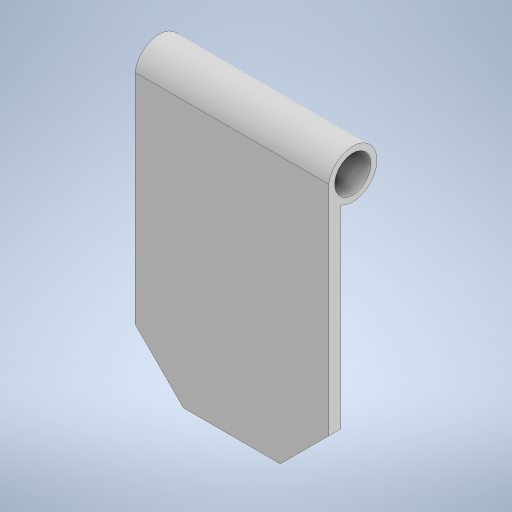
# Autodesk Inventor part: Bottom_Trava
Saved by Autodesk Inventor 2024 (Build 280153000, 153)
## iProperties
Created: 2023-11-21
Part Number: Bottom_Trava
Material: Generic
Document SubType Name: Modeling
Designer: renan
Density: 1 g/cm^3
Appearance: Default
Author: renan
Autodesk Inventor part; units mm, degrees
ref_plane "YZ Plane" through (0, 0, 0) normal (1, 0, 0) x (0, 1, 0)
ref_plane "XZ Plane" through (0, 0, 0) normal (0, 1, 0) x (-1, 0, 0)
ref_plane "XY Plane" through (0, 0, 0) normal (0, 0, 1) x (1, 0, 0)
sketch "Sketch1" plane through (0, 0, 0) normal (0, 0, 1) x (1, 0, 0)
  line L0 (0, 0) -> (-8, 0)
  line L1 (-8, 0) -> (-8, 10)
  line L2 (-8, 10) -> (0, 10)
  line L3 (0, 10) -> (0, 0)
  dimension "d2" = 10
  dimension "d3" = 8
  constraints: 8 end point, 2 parallel, 1 horizontal, 1 perpendicular
  measures "d2" distance of L0.end L1.end
  measures "d3" distance of L1.end L2.end
extrude "Extrusion1" add sketch "Sketch1" along normal blind 0.5
sketch "Sketch2" plane through (0, 0, 0) normal (1, 0, 0) x (0, 0, -1)
  line L0 (-0.5, 10) -> (-0.5, 11)
  arc A0 (0, 10) -> (-0.5, 11) centre (0.4916, 10.8708) ccw
  line L1 (0, 10) -> (-0.5, 10) projected
  line L2 (0, 10) -> (-0.5, 10)
  point P0 (0, 0)
  dimension "d4" = 1
  dimension "d5" = 1
  constraints: 4 end point, 2 point on circle, 1 centre point, 1 collinear, 1 vertical
  measures "d4" distance of L0.start L0.end
  measures "d5" radius of A0
extrude "Extrusion2" add sketch "Sketch2" against normal blind 8
sketch "Sketch3" plane through (0, 0, 0.5) normal (1, 0, 0) x (0, 0, -1)
  arc A0 (0.5, 10) -> (0, 11) centre (0.9916, 10.8708) ccw projected
  circle A1 centre (0.9916, 10.8708) radius 0.75
  point P0 (0.5, 0)
  dimension "d8" = 1.5
  constraints: 1 centre point, 1 coincident
  measures "d8" diameter of A1
extrude "Extrusion3" cut sketch "Sketch3" against normal blind 8
chamfer "Chamfer1" distance 2 angle 45 2 edges at (-8, 0, 0.25) (0, 0, 0.25)
body "Solid1"
